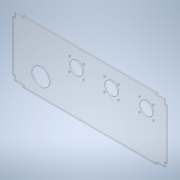
# Autodesk Inventor part: 103.015.01_Abdeckung_Gestell_oben
Saved by Autodesk Inventor 2021 (Build 250183000, 183)
## iProperties
Created: 2021-11-25
Part Number: 103.015.01_Abdeckung_Gestell_oben
Material: PMMA-Kunststoff
Document SubType Name: Modeling
Designer: Sebastian Seewald
Mass: 65.5279 g
Surface Area: 298.591 cm^2
Volume: 55.1582 cm^3
Density: 1.188 g/cm^3
Appearance: Polycarbonat - klar
Author: Sebastian Seewald
Autodesk Inventor part; units mm, degrees
ref_plane "YZ Plane" through (0, 0, 0) normal (1, 0, 0) x (0, 1, 0)
ref_plane "XZ Plane" through (0, 0, 0) normal (0, 1, 0) x (-1, 0, 0)
ref_plane "XY Plane" through (0, 0, 0) normal (0, 0, 1) x (1, 0, 0)
sketch "Skizze1" plane through (0, 0, 0) normal (0, 0, 1) x (1, 0, 0)
  line L0 (0, 0) -> (526.5, 0)
  line L1 (526.5, 0) -> (526.5, 212.5)
  line L2 (526.5, 212.5) -> (0, 212.5)
  line L3 (0, 212.5) -> (0, 0)
  line L4 (0, 212.5) -> (35, 212.5)
  line L5 (35, 212.5) -> (35, 206.15)
  line L6 (35, 206.15) -> (0, 206.15)
  line L7 (0, 206.15) -> (0, 212.5)
  line L8 (0, 212.5) -> (6.35, 212.5)
  line L9 (6.35, 212.5) -> (6.35, 192.5)
  line L10 (6.35, 192.5) -> (0, 192.5)
  line L11 (0, 192.5) -> (0, 212.5)
  line L12 (0, 106.25) -> (526.5, 106.25) construction
  line L13 (263.25, 212.5) -> (263.25, 0) construction
  line L14 (0, 0) -> (35, 0)
  line L15 (35, 0) -> (35, 6.35)
  line L16 (35, 6.35) -> (0, 6.35)
  line L17 (0, 6.35) -> (0, 0)
  line L18 (0, 0) -> (6.35, 0)
  line L19 (6.35, 0) -> (6.35, 20)
  line L20 (6.35, 20) -> (0, 20)
  line L21 (0, 20) -> (0, 0)
  line L22 (526.5, 212.5) -> (526.5, 0)
  line L23 (526.5, 212.5) -> (491.5, 212.5)
  line L24 (491.5, 212.5) -> (491.5, 206.15)
  line L25 (491.5, 206.15) -> (526.5, 206.15)
  line L26 (526.5, 206.15) -> (526.5, 212.5)
  line L27 (526.5, 212.5) -> (520.15, 212.5)
  line L28 (520.15, 212.5) -> (520.15, 192.5)
  line L29 (520.15, 192.5) -> (526.5, 192.5)
  line L30 (526.5, 192.5) -> (526.5, 212.5)
  line L31 (526.5, 0) -> (520.15, 0)
  line L32 (526.5, 0) -> (491.5, 0)
  line L33 (491.5, 0) -> (491.5, 6.35)
  line L34 (491.5, 6.35) -> (526.5, 6.35)
  line L35 (520.15, 0) -> (520.15, 20)
  line L36 (526.5, 6.35) -> (526.5, 0)
  line L37 (520.15, 20) -> (526.5, 20)
  line L38 (526.5, 20) -> (526.5, 0)
  point P0 (526.5, 192.5)
  point P1 (520.15, 206.15)
  point P2 (491.5, 212.5)
  point P3 (6.35, 206.15)
  point P4 (0, 192.5)
  point P5 (0, 20)
  point P6 (6.35, 6.35)
  point P7 (491.5, 0)
  point P8 (520.15, 6.35)
  point P9 (526.5, 20)
  dimension "d0" = 526.5
  dimension "d1" = 212.5
  dimension "d2" = 35
  dimension "d3" = 6.35
  dimension "d4" = 6.35
  dimension "d5" = 20
  constraints: 78 end point, 18 symmetric about line, 6 parallel, 4 midpoint, 3 horizontal, 3 perpendicular
  measures "d0" distance of L1.end L2.end
  measures "d1" distance between parallel lines of L0 L2
  measures "d2" distance between parallel lines of L3 L5
  measures "d3" distance between parallel lines of L2 L6
  measures "d4" distance between parallel lines of L3 L9
  measures "d5" distance between parallel lines of L2 L10
extrude "Extrusion1" add sketch "Skizze1" along normal blind 4 contours L15 L16 L19 L20 L3 L10 L9 L6 L5 L2 L24 L25 L28 L29 L1 L37 L35 L34 L33 L0
sketch "Skizze3" plane through (0, 0, 4) normal (0, 0, 1) x (1, 0, 0)
  circle A0 centre (217.25, 148.65) radius 22.5
  circle A1 centre (337.25, 148.65) radius 22.5
  circle A2 centre (457.25, 148.65) radius 22.5
  circle A3 centre (95.35, 61.35) radius 30
  line L0 (520.15, 206.15) -> (491.5, 206.15) projected
  line L1 (520.15, 192.5) -> (520.15, 206.15) projected
  line L2 (6.35, 20) -> (6.35, 6.35) projected
  line L3 (6.35, 6.35) -> (35, 6.35) projected
  point P0 (0, 0)
  dimension "d19" = 45
  dimension "d20" = 45
  dimension "d21" = 45
  dimension "d22" = 60
  dimension "d23" = 120
  dimension "d24" = 120
  dimension "d25" = 57.5
  dimension "d26" = 62.9
  dimension "d27" = 89
  dimension "d28" = 55
  constraints: 4 centre point, 2 horizontal alignment
  measures "d19" diameter of A0
  measures "d20" diameter of A1
  measures "d21" diameter of A2
  measures "d22" diameter of A3
  measures "d23" distance of A1.centre A0.centre
  measures "d24" distance of A2.centre A1.centre
  measures "d25" distance from line of L0 A1.centre
  measures "d26" distance from line of L1 A2.centre
  measures "d27" distance from line of L2 A3.centre
  measures "d28" distance from line of L3 A3.centre
extrude "Extrusion3" cut sketch "Skizze3" against normal blind 10
sketch "Skizze4" plane through (0, 0, 4) normal (0, 0, 1) x (1, 0, 0)
  circle A0 centre (193.25, 171.1) radius 2.6
  circle A1 centre (241.25, 171.1) radius 2.6
  circle A2 centre (241.25, 124.85) radius 2.6
  circle A3 centre (193.25, 124.85) radius 2.6
  circle A4 centre (217.25, 148.65) radius 22.5 projected
  line L0 (491.5, 212.5) -> (35, 212.5) projected
  line L1 (277.25, 212.5) -> (277.25, 70.6491) construction
  line L2 (397.25, 212.5) -> (397.25, 70.6491) construction
  circle A5 centre (337.25, 148.65) radius 22.5 projected
  circle A6 centre (361.25, 171.1) radius 2.6
  circle A7 centre (313.25, 171.1) radius 2.6
  circle A8 centre (313.25, 124.85) radius 2.6
  circle A9 centre (361.25, 124.85) radius 2.6
  circle A10 centre (481.25, 171.1) radius 2.6
  circle A11 centre (481.25, 124.85) radius 2.6
  circle A12 centre (433.25, 171.1) radius 2.6
  circle A13 centre (433.25, 124.85) radius 2.6
  point P0 (0, 0)
  point P1 (337.25, 148.65)
  point P2 (457.25, 148.65)
  point P3 (457.25, 148.65)
  dimension "d31" = 5.2
  dimension "d32" = 5.2
  dimension "d33" = 5.2
  dimension "d34" = 5.2
  dimension "d35" = 48
  dimension "d36" = 46.25
  dimension "d37" = 24
  dimension "d38" = 24
  dimension "d39" = 22.45
  dimension "d40" = 23.8
  dimension "d43" = 60
  dimension "d44" = 60
  constraints: 12 centre point, 11 symmetric about line, 4 end point, 2 horizontal alignment, 2 point on line, 2 vertical, 2 vertical alignment, 8 other
  measures "d31" diameter of A0
  measures "d32" diameter of A1
  measures "d33" diameter of A2
  measures "d34" diameter of A3
  measures "d35" distance of A1.centre A0.centre
  measures "d36" distance of A3.centre A0.centre
  measures "d37" horizontal distance of A4.centre A0.centre
  measures "d38" horizontal distance of A4.centre A1.centre
  measures "d39" vertical distance of A4.centre A0.centre
  measures "d40" vertical distance of A3.centre A4.centre
  measures "d43" distance from line of A4.centre L1
  measures "d44" distance from line of A5.centre L2
extrude "Extrusion4" cut sketch "Skizze4" against normal blind 10 contours A0 | A1 | A2 | A3 | A6 | A7 | A8 | A9 | A10 | A11 | A12 | A13
